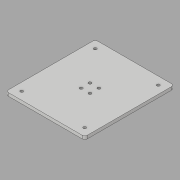
# Autodesk Inventor part: B_base 1
Saved by Autodesk Inventor 2019 (Build 230136000, 136)
## iProperties
Created: 2021-11-05
Part Number: B_base 1
Material: Generic
Document SubType Name: Modeling
Designer: Mohamed
Density: 1 g/cm^3
Appearance: Default
Author: Mohamed
Autodesk Inventor part; units mm, degrees
ref_plane "YZ Plane" through (0, 0, 0) normal (1, 0, 0) x (0, 1, 0)
ref_plane "XZ Plane" through (0, 0, 0) normal (0, 1, 0) x (-1, 0, 0)
ref_plane "XY Plane" through (0, 0, 0) normal (0, 0, 1) x (1, 0, 0)
sketch "Sketch1" plane through (0, 0, 0) normal (0, 1, 0) x (-1, 0, 0)
  line L0 (5, 0) -> (145, 0)
  line L1 (150, -5) -> (150, -165)
  line L2 (145, -170) -> (5, -170)
  line L3 (0, -165) -> (0, -5)
  arc A0 (150, -5) -> (145, 0) centre (145, -5) ccw
  arc A1 (145, -170) -> (150, -165) centre (145, -165) ccw
  arc A2 (5, 0) -> (0, -5) centre (5, -5) ccw
  arc A3 (0, -165) -> (5, -170) centre (5, -165) ccw
  circle A4 centre (135, -155) radius 2.75
  circle A5 centre (15, -155) radius 2.75
  circle A6 centre (15, -15) radius 2.75
  circle A7 centre (135, -15) radius 2.75
  line L4 (75, -85) -> (87, -85) construction
  circle A8 centre (66.4666, -93.5334) radius 2.75
  circle A9 centre (83.0375, -93.9106) radius 2.75
  circle A10 centre (83.4853, -76.5147) radius 2.75
  circle A11 centre (66.9625, -76.0894) radius 2.75
  point P0 (0, 0)
  point P1 (150, -170)
  point P2 (150, 0)
  point P3 (0, -170)
  dimension "d0" = 150
  dimension "d1" = 170
  dimension "d2" = 5
  dimension "d7" = 5.5
  dimension "d11" = 5.5
  dimension "d12" = 5.5
  dimension "d13" = 5.5
  dimension "d19" = 5.5
  dimension "d20" = 5.5
  dimension "d21" = 5.5
  dimension "d22" = 5.5
  constraints: 12 centre point, 10 end point, 8 point on circle, 8 point on line, 8 tangent, 3 equal radius, 2 horizontal, 2 parallel, 1 perpendicular
  measures "d0" distance of point (150, -170) point (0, -170)
  measures "d1" distance of point (150, 0) point (150, -170)
  measures "d2" radius of A0
  measures "d7" diameter of A4
  measures "d11" diameter of A5
  measures "d12" diameter of A6
  measures "d13" diameter of A7
  measures "d19" diameter of A8
  measures "d20" diameter of A9
  measures "d21" diameter of A10
  measures "d22" diameter of A11
extrude "Extrusion1" add sketch "Sketch1" along normal blind 6 contours L0 A0 L1 A1 L2 A3 L3 A2 | A4 | A5 | A6 | A7 | A8 | A9 | A10 | A11
sketch "Sketch2" plane through (0, 6, 0) normal (0, 1, 0) x (1, 0, 0)
  line L0 (-150, 165) -> (-150, 5) projected
  line L1 (0, 5) -> (0, 165) projected
  line L2 (0, 15) -> (15, 15) construction
  line L3 (-5, 170) -> (-145, 170) projected
  line L4 (-15, 170) -> (0, 170) construction
  circle A0 centre (-135, 155) radius 2.75
  circle A1 centre (-15, 155) radius 2.75
  circle A2 centre (-15, 15) radius 2.75
  circle A3 centre (-135, 15) radius 2.75
  line L5 (-75, 85) -> (-63, 85) construction
  circle A4 centre (-66.5147, 93.4853) radius 2.75
  circle A5 centre (-83.4853, 93.4853) radius 2.75
  circle A6 centre (-83.4853, 76.5147) radius 2.75
  circle A7 centre (-66.5147, 76.5147) radius 2.75
  point P0 (0, 0)
  dimension "d30" = 5.5
  dimension "d31" = 5.5
  dimension "d32" = 5.5
  dimension "d33" = 5.5
  dimension "d40" = 5.5
  dimension "d41" = 5.5
  dimension "d42" = 5.5
  dimension "d43" = 5.5
  constraints: 8 centre point, 6 end point, 3 horizontal, 2 point on line
  measures "d30" diameter of A0
  measures "d31" diameter of A1
  measures "d32" diameter of A2
  measures "d33" diameter of A3
  measures "d40" diameter of A4
  measures "d41" diameter of A5
  measures "d42" diameter of A6
  measures "d43" diameter of A7
extrude "Extrusion2" cut sketch "Sketch2" against normal blind 6
body "Solid1"
